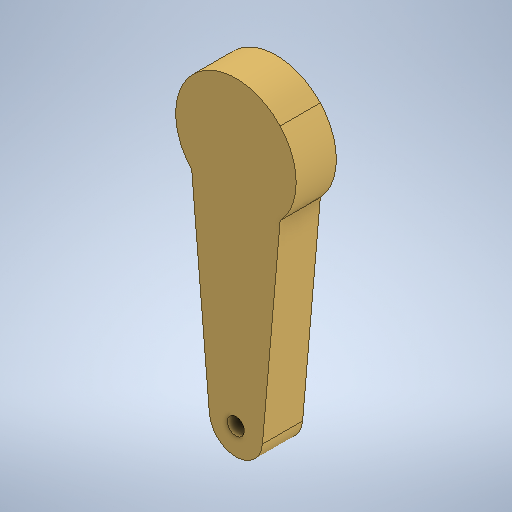
# Autodesk Inventor part: HornProfile
Saved by Autodesk Inventor 2025.1 (Build 291241000, 241)
## iProperties
Created: 2024-11-17
Part Number: HornProfile
Material: Generic
Document SubType Name: Modeling
Designer: 13156
Density: 1 g/cm^3
Appearance: Default
Author: 13156
Autodesk Inventor part; units mm, degrees
ref_plane "YZ Plane" through (0, 0, 0) normal (1, 0, 0) x (0, 1, 0)
ref_plane "XZ Plane" through (0, 0, 0) normal (0, 1, 0) x (-1, 0, 0)
ref_plane "XY Plane" through (0, 0, 0) normal (0, 0, 1) x (1, 0, 0)
sketch "Sketch3" plane through (0, 0, 0) normal (0, 0, 1) x (1, 0, 0)
  circle A0 centre (0, 24) radius 0.85
  circle A1 centre (0, -24) radius 0.85
  line L0 (0, 0) -> (0, 24) construction
  line L1 (0, -24) -> (0, 0) construction
  circle A2 centre (0, 24) radius 2.65
  circle A3 centre (0, -24) radius 2.65
  circle A4 centre (0, 0) radius 6
  line L2 (-2.6399, -24.2306) -> (-4.4, -4.0792)
  line L3 (4.4, -4.0792) -> (2.6399, -24.2306)
  line L4 (-4.4, 4.0792) -> (-2.6399, 24.2306)
  line L5 (2.6399, 24.2306) -> (4.4, 4.0792)
  circle A5 centre (0, 0) radius 1.5
  circle A6 centre (0, 0) radius 4
  dimension "d0" = 1.7
  dimension "d1" = 1.7
  dimension "d2" = 24
  dimension "d3" = 5.3
  dimension "d4" = 5.3
  dimension "d5" = 12
  dimension "d6" = 8.8
  dimension "d7" = 8.8
  dimension "d8" = 3
  dimension "d9" = 8
  constraints: 12 end point, 8 point on circle, 7 centre point, 5 coincident, 4 tangent, 3 equal length, 1 collinear, 1 vertical
  measures "d0" diameter of A1
  measures "d1" diameter of A0
  measures "d2" distance of L0.start L0.end
  measures "d3" diameter of A2
  measures "d4" diameter of A3
  measures "d5" diameter of A4
  measures "d6" distance of L5.end L4.start
  measures "d7" distance of L3.start L2.end
  measures "d8" diameter of A5
  measures "d9" diameter of A6
extrude "Extrusion1" add sketch "Sketch3" along normal blind 4 contours A2 | A2 L5 A4 L4 | A4 | A4 L3 A3 L2 | A3 | A5 | A6
sketch "Sketch4" plane through (0, 0, 0) normal (0, 0, -1) x (-1, 0, 0)
  line L0 (2.6399, 24.2306) -> (4.4, 4.0792) projected
  arc A0 (4.4, 4.0792) -> (-4.4, 4.0792) centre (0, -0.0053) ccw
  line L1 (-4.4, 4.0792) -> (-2.6399, 24.2306) projected
  line L2 (-4.4, 4.0792) -> (-4.7971, 27.3226)
  line L3 (-4.7971, 27.3226) -> (2.625, 27.4494)
  line L4 (2.625, 27.4494) -> (5.7014, 4.2518)
  line L5 (5.7014, 4.2518) -> (4.4, 4.0792)
  point P0 (0, 0)
  constraints: 8 end point, 2 perpendicular, 2 point on circle, 1 centre point
extrude "Extrusion2" cut sketch "Sketch4" against normal blind 10
equation "\"d4\" = d3"
equation "\"d7\" = d6"
body "Solid1"
